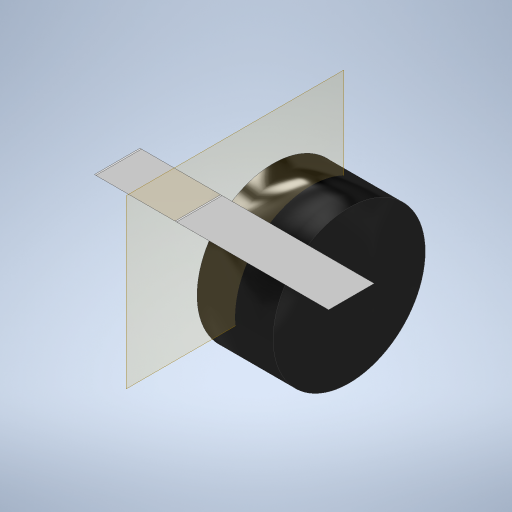
# Autodesk Inventor part: RodaP
Saved by Autodesk Inventor 2024 (Build 280153020, 153B)
## iProperties
Created: 2023-05-25
Part Number: RodaP
Material: Genérico
Document SubType Name: Modeling
Designer: victo
Density: 1 g/cm^3
Appearance: Padrão
Author: victo
Autodesk Inventor part; units mm, degrees
ref_plane "YZ Plane" through (0, 0, 0) normal (1, 0, 0) x (0, 1, 0)
ref_plane "XZ Plane" through (0, 0, 0) normal (0, 1, 0) x (-1, 0, 0)
ref_plane "XY Plane" through (0, 0, 0) normal (0, 0, 1) x (1, 0, 0)
sketch "Esboço1" plane through (0, 0, 0) normal (1, 0, 0) x (0, 1, 0)
  line L0 (0, 0) -> (-10, -9.9984)
  line L1 (-10, -9.9984) -> (-10, -12.9984)
  line L2 (-10, -12.9984) -> (0, -2.9974)
  line L3 (0, -2.9974) -> (0, 0)
  dimension "d5" = 3
  constraints: 8 end point, 1 parallel, 1 vertical
  measures "d5" distance of L0.end L1.end
extrude "Extrusão1" add sketch "Esboço1" along normal mid plane 5.4
sketch "Esboço2" plane through (-2.7, -10, -9.9984) normal (0, -0.7070505, 0.7071631) x (1, 0, 0)
  line L0 (0, 14.141) -> (0, 12.0217) projected
  line L1 (0.1, 14.141) -> (0.1, -2.1212)
  line L2 (5.3, 14.141) -> (5.3, -2.1212)
  line L3 (5.3, -2.1212) -> (0.1, -2.1212)
  line L4 (0.1, 14.141) -> (5.3, 14.141)
  point P0 (2.7, 14.141)
  point P1 (5.4, 14.141)
  constraints: 8 end point
extrude "Extrusão2" cut sketch "Esboço2" against normal blind 5.4
ref_plane "Plano de trabalho1" through (0.05, 0, 0) normal (1, 0, 0) x (0, 0, -1)
sketch "Esboço3" plane through (0.05, 0, 0) normal (1, 0, 0) x (0, 0, -1)
  line L0 (0, 0) -> (9.9984, -10) projected
  line L1 (9.9984, -10) -> (12.9984, -10) projected
  circle A0 centre (11.4984, -10) radius 5
  dimension "d14" = 10
  constraints: 1 centre point
  measures "d14" diameter of A0
extrude "Extrusão3" add sketch "Esboço3" along normal mid plane 5
